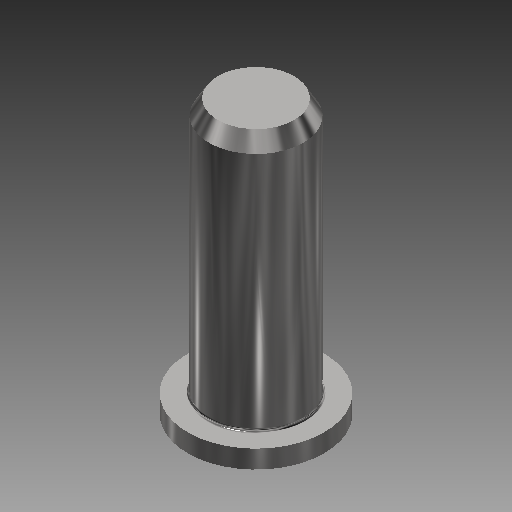
# Autodesk Inventor part: 201-03
Saved by Autodesk Inventor 2019 (Build 230136000, 136)
## iProperties
Company: Autodesk Inc.
Created: 2007-10-17
Part Number: 201-03
Document SubType Name: Modeling
Designer: Autodesk Inc.
Density: 7.85 g/cm^3
Mass: 9.37382 g
Surface Area: 7.72974 cm^2
Volume: 1.19412 cm^3
Material: Steel, High Strength Low Alloy
Description: PIVOT PIN
Appearance: Steel - Polished
Component Category: Fasteners
Author: Inventor
Autodesk Inventor part; units mm, degrees
ref_plane "YZ Plane" through (0, 0, 0) normal (1, 0, 0) x (0, 1, 0)
ref_plane "XY Plane" through (0, 0, 0) normal (0, 0, 1) x (1, 0, 0)
ref_plane "Work Plane2" through (0, 494.5349, 0) normal (0, 1, 0) x (-1, 0, 0)
sketch "Sketch1" plane through (0, 494.5349, 0) normal (0, 1, 0) x (-1, 0, 0)
  circle A0 centre (-3068.8365, 412.4332) radius 3.2
  line L0 (614.5573, 0) -> (-3687.3438, 0) projected
  line L1 (0, -83.2766) -> (0, 499.6599) projected
  circle A1 centre (-3068.8365, 412.4332) radius 3.95
  point P0 (0, 0)
  dimension "d2" = 6.4
  dimension "d3" = 412.4332
  dimension "d4" = 3068.8364
  dimension "d7" = 7.9
  constraints: 2 centre point, 1 coincident
  measures "d2" diameter of A0
  measures "d3" distance from line of L0 A0.centre
  measures "d4" distance from line of L1 A0.centre
  measures "d7" diameter of A1
extrude "Extrusion1" add sketch "Sketch1" against normal blind 21.4 contours A0 | A1
sketch "Sketch2" plane through (3068.8365, 473.1349, 412.4332) normal (0, -1, 0) x (1, 0, 0)
  circle A0 centre (0, 0) radius 3.95 projected
  circle A1 centre (0, 0) radius 5.715
  dimension "d8" = 11.43
  constraints: 1 centre point, 1 coincident
  measures "d8" diameter of A1
extrude "Extrusion2" add sketch "Sketch2" along normal blind 1.52 contours A0 | A1
fillet "Fillet1" radius 0.25 1 edges at (3072.7865, 473.1349, 412.4332)
chamfer "Chamfer2" distance 1.27 distance2 0.7554 1 edges at (3072.7865, 494.5349, 412.4332) measured on face at (3068.0463, 480.4349, 416.3034)
body "Solid1"
